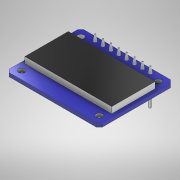
# Autodesk Inventor part: SPI_Display_0.96inch
Saved by Autodesk Inventor 2022.2 (Build 262287010, 287A)
## iProperties
Created: 2026-01-01
Part Number: SPI_Display_0.96inch
Material: Generic
Document SubType Name: Modeling
Designer: dbstj
Density: 1 g/cm^3
Appearance: 알루미늄 - 연마
Author: dbstj
Autodesk Inventor part; units mm, degrees
ref_plane "YZ Plane" through (0, 0, 0) normal (1, 0, 0) x (0, 1, 0)
ref_plane "XZ Plane" through (0, 0, 0) normal (0, 1, 0) x (-1, 0, 0)
ref_plane "XY Plane" through (0, 0, 0) normal (0, 0, 1) x (1, 0, 0)
sketch "스케치1" plane through (0, 0, 0) normal (0, 1, 0) x (-1, 0, 0)
  line L0 (15, -12) -> (-15, -12)
  line L1 (-15, -12) -> (-15, 12)
  line L2 (-15, 12) -> (15, 12)
  line L3 (15, 12) -> (15, -12)
  line L4 (15, -12) -> (-15, 12) construction
  line L5 (-15, -12) -> (15, 12) construction
  line L6 (12.5, 9.5) -> (-12.5, 9.5)
  line L7 (-12.5, 9.5) -> (-12.5, -9.5)
  line L8 (-12.5, -9.5) -> (12.5, -9.5)
  line L9 (12.5, -9.5) -> (12.5, 9.5)
  line L10 (12.5, 9.5) -> (-12.5, -9.5) construction
  line L11 (-12.5, 9.5) -> (12.5, -9.5) construction
  circle A0 centre (12.5, -9.5) radius 1
  circle A1 centre (-12.5, -9.5) radius 1
  circle A2 centre (-12.5, 9.5) radius 1
  circle A3 centre (12.5, 9.5) radius 1
  point P0 (0, 0)
  dimension "d0" = 30
  dimension "d1" = 24
  dimension "d2" = 25
  dimension "d3" = 19
  dimension "d4" = 2
  dimension "d5" = 2
  dimension "d6" = 2
  dimension "d7" = 2
  constraints: 24 end point, 4 centre point, 4 coincident, 4 midpoint, 4 parallel, 2 horizontal, 2 perpendicular
  measures "d0" distance of L1.end L2.end
  measures "d1" distance of L0.end L1.end
  measures "d2" distance of L8.end L7.end
  measures "d3" distance of L7.end L6.end
  measures "d4" diameter of A0
  measures "d5" diameter of A1
  measures "d6" diameter of A2
  measures "d7" diameter of A3
extrude "돌출1" add sketch "스케치1" along normal blind 1.2 contours L0 L1 L2 L3 | L6 A3 L9 A0 L8 A1 L7 A2
sketch "스케치2" plane through (0, 1.2, 0) normal (0, 1, 0) x (1, 0, 0)
  line L0 (-14, -7) -> (14, -7)
  line L1 (14, -7) -> (14, 7)
  line L2 (14, 7) -> (-14, 7)
  line L3 (-14, 7) -> (-14, -7)
  line L4 (-14, -7) -> (14, 7) construction
  line L5 (14, -7) -> (-14, 7) construction
  point P0 (0, 0)
  dimension "d10" = 28
  dimension "d11" = 14
  constraints: 12 end point, 2 midpoint, 2 parallel, 1 horizontal, 1 perpendicular
  measures "d10" distance of L2.end L1.end
  measures "d11" distance of L1.end L0.end
extrude "돌출2" add sketch "스케치2" along normal blind 2
sketch "스케치3" plane through (0, 1.2, 0) normal (0, 1, 0) x (1, 0, 0)
  line L0 (15, -12) -> (15, 12) projected
  line L1 (15, 12) -> (-15, 12) projected
  circle A0 centre (-8.89, 10.56) radius 0.5
  circle A1 centre (-6.35, 10.56) radius 0.5
  circle A2 centre (-3.81, 10.56) radius 0.5
  circle A3 centre (-1.27, 10.56) radius 0.5
  circle A4 centre (1.27, 10.56) radius 0.5
  circle A5 centre (3.81, 10.56) radius 0.5
  circle A6 centre (6.35, 10.56) radius 0.5
  circle A7 centre (8.89, 10.56) radius 0.5
  point P0 (0, 0)
  dimension "d14" = 2.54
  dimension "d15" = 2.54
  dimension "d16" = 2.54
  dimension "d17" = 2.54
  dimension "d18" = 2.54
  dimension "d19" = 2.54
  dimension "d20" = 2.54
  dimension "d22" = 1.44
  dimension "d23" = 1
  dimension "d24" = 1
  dimension "d25" = 1
  dimension "d26" = 1
  dimension "d27" = 1
  dimension "d28" = 1
  dimension "d29" = 1
  dimension "d53" = 1
  dimension "d113" = 13.73
  constraints: 8 centre point, 8 coincident, 7 horizontal alignment
  measures "d14" distance of point (6.35, 10.56) point (8.89, 10.56)
  measures "d15" distance of point (3.81, 10.56) point (6.35, 10.56)
  measures "d16" distance of point (1.27, 10.56) point (3.81, 10.56)
  measures "d17" distance of point (-1.27, 10.56) point (1.27, 10.56)
  measures "d18" distance of point (-3.81, 10.56) point (-1.27, 10.56)
  measures "d19" distance of point (-6.35, 10.56) point (-3.81, 10.56)
  measures "d20" distance of point (-8.89, 10.56) point (-6.35, 10.56)
  measures "d22" distance from line of L1 point (8.89, 10.56)
  measures "d23" diameter of A0
  measures "d24" diameter of A1
  measures "d25" diameter of A2
  measures "d26" diameter of A3
  measures "d27" diameter of A4
  measures "d28" diameter of A5
  measures "d29" diameter of A6
  measures "d53" diameter of A7
  measures "d113" distance from line of L0 A4.centre
extrude "돌출3" add sketch "스케치3" along normal blind 2
chamfer "모따기1" distance 0.3 distance2 2 1 edges at (5.85, 3.2, -10.56) measured on face at (6.1668, 3.2, -10.6561)
chamfer "모따기2" distance 0.3 distance2 2 1 edges at (3.31, 3.2, -10.56) measured on face at (3.8691, 3.2, -10.4042)
chamfer "모따기3" distance 0.3 distance2 2 1 edges at (0.77, 3.2, -10.56) measured on face at (1.1007, 3.2, -10.7255)
chamfer "모따기4" distance 0.3 distance2 2 1 edges at (-1.77, 3.2, -10.56) measured on face at (-1.4393, 3.2, -10.7255)
chamfer "모따기5" distance 0.3 distance2 2 1 edges at (-4.31, 3.2, -10.56) measured on face at (-3.8038, 3.2, -10.4639)
chamfer "모따기6" distance 0.3 distance2 2 1 edges at (-6.85, 3.2, -10.56) measured on face at (-6.4319, 3.2, -10.5921)
chamfer "모따기7" distance 0.3 distance2 2 1 edges at (-9.39, 3.2, -10.56) measured on face at (-9.0639, 3.2, -10.4132)
chamfer "모따기8" distance 0.3 distance2 2 1 edges at (8.39, 3.2, -10.56) measured on face at (9.0549, 3.2, -10.6705)
sketch "스케치4" plane through (0, 0, 0) normal (0, -1, 0) x (1, 0, 0)
  circle A0 centre (6.35, -10.56) radius 0.5 projected
  circle A1 centre (3.81, -10.56) radius 0.5 projected
  circle A2 centre (1.27, -10.56) radius 0.5 projected
  circle A3 centre (-1.27, -10.56) radius 0.5 projected
  circle A4 centre (-3.81, -10.56) radius 0.5 projected
  circle A5 centre (-6.35, -10.56) radius 0.5 projected
  circle A6 centre (-8.89, -10.56) radius 0.5 projected
  circle A7 centre (8.89, -10.56) radius 0.5 projected
  line L0 (10.41, -11.83) -> (-10.41, -11.83)
  line L1 (-10.41, -11.83) -> (-10.41, -9.29)
  line L2 (-10.41, -9.29) -> (10.41, -9.29)
  line L3 (10.41, -9.29) -> (10.41, -11.83)
  point P0 (0, 0)
  dimension "d57" = 20.82
  dimension "d58" = 2.54
  dimension "d59" = 1.52
  dimension "d60" = 1.27
  constraints: 8 end point, 2 parallel, 1 horizontal, 1 perpendicular
  measures "d57" distance of L1.end L2.end
  measures "d58" distance of L0.end L1.end
  measures "d59" distance from line of L3 A7.centre
  measures "d60" distance from line of L0 A7.centre
extrude "돌출4" add sketch "스케치4" along normal blind 2.5 contours A0 | A1 | A2 | A3 | A4 | A5 | A6 | A7 | L0 L1 L2 L3
sketch "스케치5" plane through (0, -2.5, 0) normal (0, -1, 0) x (1, 0, 0)
  circle A0 centre (8.89, -10.56) radius 0.5 projected
  circle A1 centre (6.35, -10.56) radius 0.5 projected
  circle A2 centre (3.81, -10.56) radius 0.5 projected
  circle A3 centre (1.27, -10.56) radius 0.5 projected
  circle A4 centre (-1.27, -10.56) radius 0.5 projected
  circle A5 centre (-3.81, -10.56) radius 0.5 projected
  circle A6 centre (-6.35, -10.56) radius 0.5 projected
  circle A7 centre (-8.89, -10.56) radius 0.5 projected
  line L0 (9.09, -10.86) -> (8.49, -10.86)
  line L1 (8.49, -10.86) -> (8.49, -10.26)
  line L2 (8.49, -10.26) -> (9.09, -10.26)
  line L3 (9.09, -10.26) -> (9.09, -10.86)
  line L4 (9.09, -10.86) -> (8.49, -10.26) construction
  line L5 (8.49, -10.86) -> (9.09, -10.26) construction
  line L6 (6.55, -10.86) -> (5.95, -10.86)
  line L7 (6.55, -10.26) -> (6.55, -10.86)
  line L8 (5.95, -10.26) -> (6.55, -10.26)
  line L9 (5.95, -10.86) -> (5.95, -10.26)
  line L10 (4.01, -10.86) -> (3.41, -10.86)
  line L11 (4.01, -10.26) -> (4.01, -10.86)
  line L12 (3.41, -10.26) -> (4.01, -10.26)
  line L13 (3.41, -10.86) -> (3.41, -10.26)
  line L14 (1.47, -10.86) -> (0.87, -10.86)
  line L15 (1.47, -10.26) -> (1.47, -10.86)
  line L16 (0.87, -10.26) -> (1.47, -10.26)
  line L17 (0.87, -10.86) -> (0.87, -10.26)
  line L18 (-1.07, -10.86) -> (-1.67, -10.86)
  line L19 (-1.07, -10.26) -> (-1.07, -10.86)
  line L20 (-1.67, -10.26) -> (-1.07, -10.26)
  line L21 (-1.67, -10.86) -> (-1.67, -10.26)
  line L22 (-3.61, -10.86) -> (-4.21, -10.86)
  line L23 (-3.61, -10.26) -> (-3.61, -10.86)
  line L24 (-4.21, -10.26) -> (-3.61, -10.26)
  line L25 (-4.21, -10.86) -> (-4.21, -10.26)
  line L26 (-6.15, -10.86) -> (-6.75, -10.86)
  line L27 (-6.15, -10.26) -> (-6.15, -10.86)
  line L28 (-6.75, -10.26) -> (-6.15, -10.26)
  line L29 (-6.75, -10.86) -> (-6.75, -10.26)
  line L30 (-8.69, -10.86) -> (-9.29, -10.86)
  line L31 (-8.69, -10.26) -> (-8.69, -10.86)
  line L32 (-9.29, -10.26) -> (-8.69, -10.26)
  line L33 (-9.29, -10.86) -> (-9.29, -10.26)
  point P0 (0, 0)
  point P1 (8.79, -10.56)
  point P2 (-1.27, -10.56)
  point P3 (-3.81, -10.56)
  point P4 (-6.35, -10.56)
  point P5 (-8.89, -10.56)
  dimension "d63" = 0.6
  dimension "d64" = 0.6
  dimension "d67" = 2.54
  constraints: 68 end point, 2 horizontal, 2 midpoint, 2 parallel, 1 collinear, 1 perpendicular, 62 other
  measures "d63" distance of L1.end L2.end
  measures "d64" distance of L0.end L1.end
  measures "d67" distance of L0.start L6.start
extrude "돌출5" add sketch "스케치5" along normal blind 6 contours L2 L3 L0 L1 | L8 L7 L6 L9 | L12 L11 L10 L13 | L16 L15 L14 L17 | L20 L19 L18 L21 | L24 L23 L22 L25 | L28 L27 L26 L29 | L32 L31 L30 L33
chamfer "모따기9" distance 0.15 angle 45 32 edges at (8.79, -8.5, -10.86) (8.49, -8.5, -10.56) (8.79, -8.5, -10.26) (9.09, -8.5, -10.56) (6.25, -8.5, -10.86) (6.55, -8.5, -10.56) (6.25, -8.5, -10.26) (5.95, -8.5, -10.56) (3.71, -8.5, -10.86) (3.41, -8.5, -10.56) (3.71, -8.5, -10.26) (4.01, -8.5, -10.56) (1.17, -8.5, -10.26) (0.87, -8.5, -10.56) (1.17, -8.5, -10.86) (1.47, -8.5, -10.56) (-1.37, -8.5, -10.86) (-1.07, -8.5, -10.56) (-1.37, -8.5, -10.26) (-1.67, -8.5, -10.56) (-3.91, -8.5, -10.86) (-3.61, -8.5, -10.56) (-3.91, -8.5, -10.26) (-4.21, -8.5, -10.56) (-6.15, -8.5, -10.56) (-6.45, -8.5, -10.86) (-6.75, -8.5, -10.56) (-6.45, -8.5, -10.26) (-8.99, -8.5, -10.86) (-8.69, -8.5, -10.56) (-8.99, -8.5, -10.26) (-9.29, -8.5, -10.56)
chamfer "모따기10" distance 1 angle 45 4 edges at (15, 0.6, -12) (15, 0.6, 12) (-15, 0.6, 12) (-15, 0.6, -12)
equation "\"d5\" = d4"
equation "\"d6\" = d4"
equation "\"d7\" = d4"
equation "\"d15\" = d14"
equation "\"d16\" = d14"
equation "\"d17\" = d14"
equation "\"d18\" = d14"
equation "\"d19\" = d14"
equation "\"d20\" = d14"
